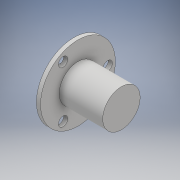
# Autodesk Inventor part: SlipRing-022A-12
Saved by Autodesk Inventor 2017 (Build 210142000, 142)
## iProperties
Created: 2017-04-28
Part Number: SlipRing-022A-12
Material: Generic
Document SubType Name: Modeling
Designer: s4321966
Density: 1 g/cm^3
Appearance: Default
Author: s4321966
Autodesk Inventor part; units mm, degrees
ref_plane "YZ Plane" through (0, 0, 0) normal (1, 0, 0) x (0, 1, 0)
ref_plane "XZ Plane" through (0, 0, 0) normal (0, 1, 0) x (-1, 0, 0)
ref_plane "XY Plane" through (0, 0, 0) normal (0, 0, 1) x (1, 0, 0)
sketch "Sketch1" plane through (0, 0, 0) normal (1, 0, 0) x (0, 1, 0)
  circle A0 centre (0, 0) radius 22
  dimension "d0" = 44
  constraints: 1 centre point, 1 coincident
  measures "d0" diameter of A0
extrude "Extrusion1" add sketch "Sketch1" along normal blind 2.4
sketch "Sketch2" plane through (2.4, 0, 0) normal (1, 0, 0) x (0, 0, -1)
  line L0 (0, 0) -> (0, 17.5)
  circle A0 centre (0, 17.5) radius 2.75
  circle A1 centre (-15.1554, -8.75) radius 2.75
  circle A2 centre (15.1554, -8.75) radius 2.75
  dimension "d3" = 17.5
  dimension "d4" = 5.5
  dimension "d7" = 360
  constraints: 3 centre point, 2 end point, 1 coincident, 1 vertical, 7 other
  measures "d3" distance of L0.start L0.end
  measures "d4" diameter of A0
extrude "Extrusion2" cut sketch "Sketch2" against normal blind 2.4
sketch "Sketch3" plane through (2.4, 0, 0) normal (1, 0, 0) x (0, 0, -1)
  circle A0 centre (0, 0) radius 11
  dimension "d11" = 22
  constraints: 1 centre point, 1 coincident
  measures "d11" diameter of A0
extrude "Extrusion3" add sketch "Sketch3" along normal blind 25.6
sketch "Sketch4" plane through (0, 0, 0) normal (-1, 0, 0) x (0, 0, 1)
  circle A0 centre (0, 0) radius 11 projected
  circle A1 centre (0, 0) radius 3.9
  dimension "d14" = 7.8
  constraints: 1 centre point, 1 coincident
  measures "d14" diameter of A1
extrude "Extrusion4" add sketch "Sketch4" along normal blind 9 contours A1
body "Solid1"
